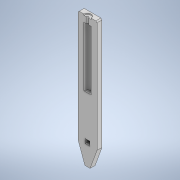
# Autodesk Inventor part: graduated_foot_03
Saved by Autodesk Inventor 2020 (Build 240168000, 168)
## iProperties
Created: 2019-12-19
Part Number: graduated_foot_03
Material: Générique
Document SubType Name: Modeling
Designer: damien
Density: 1 g/cm^3
Appearance: Par défaut
Author: damien
Autodesk Inventor part; units mm, degrees
ref_plane "YZ Plane" through (0, 0, 0) normal (1, 0, 0) x (0, 1, 0)
ref_plane "XZ Plane" through (0, 0, 0) normal (0, 1, 0) x (-1, 0, 0)
ref_plane "XY Plane" through (0, 0, 0) normal (0, 0, 1) x (1, 0, 0)
sketch "Esquisse1" plane through (0, 0, 0) normal (0, 0, 1) x (1, 0, 0)
  line L0 (0, 0) -> (80, 0)
  line L1 (80, 0) -> (80, 550)
  line L2 (80, 550) -> (0, 550)
  line L3 (0, 550) -> (0, 0)
  dimension "d0" = 80
  dimension "d1" = 550
  constraints: 8 end point, 2 parallel, 1 horizontal, 1 perpendicular
  measures "d0" distance of L0.start L0.end
  measures "d1" distance of L2.end L0.start
extrude "Extrusion1" add sketch "Esquisse1" along normal blind 21
chamfer "Chanfrein1" distance 5 angle 45 2 edges at (0, 550, 10.5) (80, 550, 10.5)
sketch "Esquisse4" plane through (0, 0, 21) normal (0, 0, 1) x (1, 0, 0)
  line L0 (0, 545) -> (0, 0) projected
  line L1 (80, 0) -> (80, 545) projected
  line L2 (0, 80) -> (29.1176, 0)
  line L3 (0, 0) -> (80, 0) projected
  line L4 (50.8824, 0) -> (80, 80)
  line L5 (29.1176, 0) -> (50.8824, 0)
  line L6 (30, 98.55) -> (50, 98.55)
  line L7 (50, 98.55) -> (50, 80)
  line L8 (50, 80) -> (30, 80)
  line L9 (30, 80) -> (30, 98.55)
  line L10 (40, 0) -> (40, 80) construction
  dimension "d23" = 70
  dimension "d24" = 70
  dimension "d25" = 80
  dimension "d26" = 20
  dimension "d27" = 18.55
  constraints: 16 end point, 5 point on line, 2 midpoint, 2 parallel, 1 collinear, 1 equal length, 1 horizontal, 1 perpendicular, 1 vertical
  measures "d23" angle of L3 L2
  measures "d24" angle of L3 L4
  measures "d25" distance from line of L3 L2.start
  measures "d26" distance of L7.end L8.end
  measures "d27" distance of L6.end L7.end
extrude "Extrusion3" cut sketch "Esquisse4" against normal blind 21
sketch "Esquisse6" plane through (0, 0, 21) normal (0, 0, 1) x (1, 0, 0)
  line L0 (75, 550) -> (5, 550) construction
  line L1 (35, 520) -> (35, 545)
  line L2 (0, 545) -> (0, 80) construction
  line L3 (0, 535) -> (35, 535) construction
  line L4 (45, 535) -> (80, 535) construction
  line L5 (80, 80) -> (80, 545) construction
  line L6 (25, 270) -> (25, 520)
  line L7 (25, 520) -> (35, 520)
  line L8 (25, 395) -> (0, 395) construction
  line L9 (55, 395) -> (80, 395) construction
  line L10 (40, 550) -> (40, 270) construction
  line L11 (25, 270) -> (40, 270)
  line L12 (40, 270) -> (40, 550)
  line L13 (35, 545) -> (25, 545)
  line L14 (25, 545) -> (25, 550)
  line L15 (25, 550) -> (40, 550)
  point P0 (0, 0)
  point P1 (35, 550)
  dimension "d39" = 5
  dimension "d41" = 30
  dimension "d42" = 250
  dimension "d43" = 15
  dimension "d45" = 5
  dimension "d46" = 15
  constraints: 26 end point, 9 point on line, 6 horizontal, 3 collinear, 2 midpoint, 2 perpendicular, 2 vertical
  measures "d39" distance between parallel lines of L10 L1
  measures "d41" distance of L1.start point (35, 550)
  measures "d42" distance of L6.start L6.end
  measures "d43" distance of L6.start L10.end
  measures "d45" distance of L13.end L14.end
  measures "d46" distance between parallel lines of L10 L14
revolve "Révolution1" cut sketch "Esquisse6" angle 360 about axis through (40, 550, 21) along (0, -1, 0)
